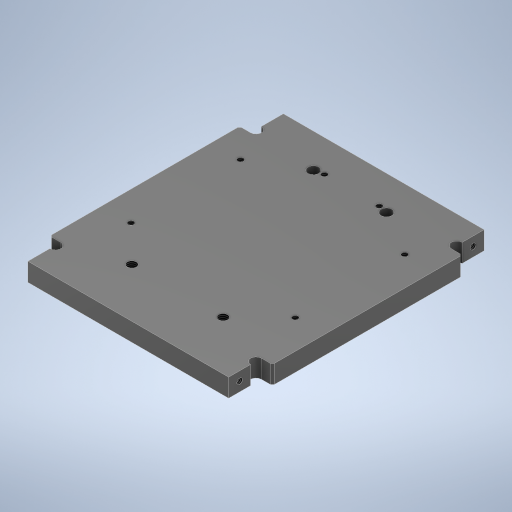
# Autodesk Inventor part: HeadCircuitMountFrame
Saved by Autodesk Inventor 2024.2 (Build 282272000, 272)
## iProperties
Created: 2024-01-19
Part Number: HeadCircuitMountFrame
Material: Acetal Resin, Black
Document SubType Name: Modeling
Designer: Masato Kubotera
Density: 1.425 g/cm^3
Appearance: Smooth - Black
Mass: 11.7532 g
Surface Area: 68.8447 cm^2
Volume: 8.24788 cm^3
Vendor: meviy
Author: Masato Kubotera
Autodesk Inventor part; units mm, degrees
ref_plane "YZ Plane" through (0, 0, 0) normal (1, 0, 0) x (0, 1, 0)
ref_plane "XZ Plane" through (0, 0, 0) normal (0, 1, 0) x (-1, 0, 0)
ref_plane "XY Plane" through (0, 0, 0) normal (0, 0, 1) x (1, 0, 0)
sketch "Sketch1" plane through (0, 0, 0) normal (0, 0, 1) x (1, 0, 0)
  line L0 (35, 27.5) -> (-35, 27.5) construction
  line L1 (-35, 27.5) -> (-35, -27.5)
  line L2 (-35, -27.5) -> (35, -27.5) construction
  line L3 (35, -27.5) -> (35, 27.5)
  line L4 (35, 27.5) -> (-35, -27.5) construction
  line L5 (-35, 27.5) -> (35, -27.5) construction
  line L6 (0, 27.5) -> (0, -27.5) construction
  line L7 (35, 0) -> (-35, 0) construction
  line L8 (26, 27.5) -> (26, 30.5)
  line L9 (26, 30.5) -> (-26, 30.5)
  line L10 (-26, 30.5) -> (-26, 27.5)
  arc A0 (-29, 27.5) -> (-26, 27.5) centre (-27.5, 27.5) ccw
  line L11 (26, -27.5) -> (26, -30.5)
  line L12 (26, -30.5) -> (-26, -30.5)
  line L13 (-26, -30.5) -> (-26, -27.5)
  arc A1 (-26, -27.5) -> (-29, -27.5) centre (-27.5, -27.5) ccw
  line L14 (-32, 27.5) -> (-32, 21.5) construction
  line L15 (0, 30.5) -> (0, 27.5) construction
  line L16 (32, 27.5) -> (32, 21.5) construction
  arc A2 (26, 27.5) -> (29, 27.5) centre (27.5, 27.5) ccw
  arc A3 (29, -27.5) -> (26, -27.5) centre (27.5, -27.5) ccw
  line L17 (-17.5, -10) -> (-35, -10) construction
  line L18 (-35, -10) -> (-35, 10) construction
  line L19 (-35, 10) -> (-17.5, 10) construction
  line L20 (-17.5, 10) -> (-17.5, -10) construction
  line L21 (-17.5, -10) -> (-35, 10) construction
  line L22 (-35, -10) -> (-17.5, 10) construction
  line L23 (-26.25, -7.5) -> (-26.25, 7.5) construction
  line L24 (-25.7386, -10) -> (-25.7386, 10) construction
  circle A4 centre (-25.7386, 10) radius 2.5 construction
  line L25 (-33, 3.75) -> (-32, 3.75)
  line L26 (-30, 1.75) -> (-30, -1.75)
  line L27 (-32, -3.75) -> (-33, -3.75)
  arc A5 (-32, -3.75) -> (-30, -1.75) centre (-32, -1.75) ccw
  arc A6 (-30, 1.75) -> (-32, 3.75) centre (-32, 1.75) ccw
  arc A7 (-35, 5.75) -> (-33, 3.75) centre (-33, 5.75) ccw
  line L28 (35, -27.5) -> (29, -27.5)
  line L29 (-29, -27.5) -> (-35, -27.5)
  line L30 (-35, 27.5) -> (-29, 27.5)
  line L31 (29, 27.5) -> (35, 27.5)
  circle A8 centre (-26.25, 7.5) radius 2.5 construction
  line L32 (14.2614, -25) -> (-20.7386, -25) construction
  line L33 (-20.7386, -25) -> (-20.7386, 25) construction
  line L34 (-20.7386, 25) -> (14.2614, 25) construction
  line L35 (14.2614, 25) -> (14.2614, -25) construction
  line L36 (14.2614, -25) -> (-20.7386, 25) construction
  line L37 (-20.7386, -25) -> (14.2614, 25) construction
  line L38 (11.7614, 22.5) -> (-18.2386, 22.5) construction
  line L39 (-18.2386, 22.5) -> (-18.2386, -22.5) construction
  line L40 (-18.2386, -22.5) -> (11.7614, -22.5) construction
  line L41 (11.7614, -22.5) -> (11.7614, 22.5) construction
  line L42 (11.7614, 22.5) -> (-18.2386, -22.5) construction
  line L43 (-18.2386, 22.5) -> (11.7614, -22.5) construction
  circle A9 centre (-18.2386, 22.5) radius 2.5 construction
  arc A10 (-21.2236, 22.2) -> (-15.2536, 22.2) centre (-18.2386, 22.5) ccw
  line L44 (-21.2386, 10) -> (-21.2386, 3)
  line L45 (-13.2637, 24) -> (6.7865, 24)
  arc A11 (8.7764, 22.2) -> (14.7464, 22.2) centre (11.7614, 22.5) ccw
  arc A12 (32.802, 10.6698) -> (32.3609, 9.408) centre (46.2004, 5.2778) ccw
  line L46 (32.9466, 11.4165) -> (32.9466, 22)
  line L47 (30.9466, 24) -> (16.7363, 24)
  arc A13 (32.802, 10.6698) -> (32.9466, 11.4165) centre (30.9466, 11.4165) ccw
  line L48 (34.9466, 11.4165) -> (32.9466, 11.4165) construction
  line L49 (32.802, 8.6698) -> (32.802, 10.6698) construction
  line L50 (30.4444, 7.9799) -> (22.1342, 7.9799)
  line L51 (15.9549, 1.8007) -> (15.9549, 3)
  line L52 (13.9549, 1) -> (-19.2386, 1)
  arc A14 (30.4444, 7.9799) -> (32.3609, 9.408) centre (30.4444, 9.9799) ccw
  arc A15 (32.9466, 22) -> (30.9466, 24) centre (30.9466, 22) ccw
  arc A16 (16.7363, 24) -> (14.7464, 22.2) centre (16.7363, 22) ccw
  arc A17 (8.7764, 22.2) -> (6.7865, 24) centre (6.7865, 22) ccw
  arc A18 (-13.2637, 24) -> (-15.2536, 22.2) centre (-13.2637, 22) ccw
  arc A19 (-21.2386, 3) -> (-19.2386, 1) centre (-19.2386, 3) ccw
  arc A20 (13.9549, 1) -> (15.9549, 3) centre (13.9549, 3) ccw
  arc A21 (22.1342, 7.9799) -> (15.9549, 1.8007) centre (22.1342, 1.8007) ccw
  arc A22 (-15.2536, -22.2) -> (-21.2236, -22.2) centre (-18.2386, -22.5) ccw
  line L53 (-21.2386, -10) -> (-21.2386, -3)
  line L54 (-13.2637, -24) -> (6.7865, -24)
  arc A23 (14.7464, -22.2) -> (8.7764, -22.2) centre (11.7614, -22.5) ccw
  arc A24 (32.3609, -9.408) -> (32.802, -10.6698) centre (46.2004, -5.2778) ccw
  line L55 (32.9466, -11.4165) -> (32.9466, -22)
  line L56 (30.9466, -24) -> (16.7363, -24)
  arc A25 (32.9466, -11.4165) -> (32.802, -10.6698) centre (30.9466, -11.4165) ccw
  line L57 (30.4444, -7.9799) -> (22.1342, -7.9799)
  line L58 (15.9549, -1.8007) -> (15.9549, -3)
  line L59 (13.9549, -1) -> (-19.2386, -1)
  arc A26 (32.3609, -9.408) -> (30.4444, -7.9799) centre (30.4444, -9.9799) ccw
  arc A27 (30.9466, -24) -> (32.9466, -22) centre (30.9466, -22) ccw
  arc A28 (14.7464, -22.2) -> (16.7363, -24) centre (16.7363, -22) ccw
  arc A29 (6.7865, -24) -> (8.7764, -22.2) centre (6.7865, -22) ccw
  arc A30 (-15.2536, -22.2) -> (-13.2637, -24) centre (-13.2637, -22) ccw
  arc A31 (-19.2386, -1) -> (-21.2386, -3) centre (-19.2386, -3) ccw
  arc A32 (15.9549, -3) -> (13.9549, -1) centre (13.9549, -3) ccw
  arc A33 (15.9549, -1.8007) -> (22.1342, -7.9799) centre (22.1342, -1.8007) ccw
  line L60 (-32.9466, 13.8893) -> (-32.9466, 22)
  arc A34 (-30.9466, 24) -> (-32.9466, 22) centre (-30.9466, 22) ccw
  arc A35 (-21.2236, 22.2) -> (-23.2135, 24) centre (-23.2135, 22) ccw
  line L61 (-30.9466, 24) -> (-23.2135, 24)
  arc A36 (-21.2386, 10) -> (-29.3442, 12.6926) centre (-25.7386, 10) ccw
  arc A37 (-32.9466, 13.8893) -> (-29.3442, 12.6926) centre (-30.9466, 13.8893) ccw
  line L62 (-32.9466, -13.8893) -> (-32.9466, -22)
  arc A38 (-32.9466, -22) -> (-30.9466, -24) centre (-30.9466, -22) ccw
  line L63 (-30.9466, -24) -> (-23.2135, -24)
  arc A39 (-29.3442, -12.6926) -> (-21.2386, -10) centre (-25.7386, -10) ccw
  arc A40 (-29.3442, -12.6926) -> (-32.9466, -13.8893) centre (-30.9466, -13.8893) ccw
  arc A41 (-23.2135, -24) -> (-21.2236, -22.2) centre (-23.2135, -22) ccw
  line L64 (25, -16) -> (-25, -16) construction
  line L65 (-25, -16) -> (-25, 16) construction
  line L66 (-25, 16) -> (25, 16) construction
  line L67 (25, 16) -> (25, -16) construction
  line L68 (25, -16) -> (-25, 16) construction
  line L69 (-25, -16) -> (25, 16) construction
  line L70 (21.5, -12.5) -> (21.5, 12.5) construction
  point P0 (0, 0)
  point P1 (0, 0)
  point P2 (0, -0.0008)
  point P3 (-29, -27.5)
  point P4 (26, -27.5)
  point P5 (-26, -27.5)
  point P6 (-26, -27.5)
  point P7 (26, -27.5)
  point P8 (-26.25, 0)
  point P9 (29, -27.5)
  point P10 (29, -10)
  point P11 (-3.2386, 0)
  point P12 (-21.2386, 22.5)
  point P13 (-15.6405, 24)
  point P14 (9.1633, 24)
  point P15 (14.3595, 24)
  point P16 (32.0128, 7.9799)
  point P17 (0, 0)
  dimension "d19" = 3
  dimension "d20" = 52
  dimension "d37" = 55
  dimension "d40" = 6
  dimension "d41" = 6
  dimension "d59" = 70
  dimension "d60" = 1.5
  dimension "d61" = 17.5
  dimension "d62" = 20
  dimension "d63" = 15
  dimension "d90" = 20
  dimension "d98" = 5
  dimension "d100" = 7.5
  dimension "d101" = 5
  dimension "d111" = 5
  dimension "d113" = 50
  dimension "d114" = 35
  dimension "d115" = 5
  dimension "d117" = 5
  dimension "d118" = 2
  dimension "d119" = 2
  dimension "d120" = 2
  dimension "d124" = 2
  dimension "d125" = 2
  dimension "d126" = 3
  dimension "d128" = 50
  dimension "d129" = 32
  dimension "d130" = 25
  dimension "d131" = 3.5
  dimension "d140" = 0
  dimension "d141" = 10
  constraints: 140 end point, 83 point on circle, 60 symmetric about line, 42 centre point, 30 tangent, 18 midpoint, 14 coincident, 14 horizontal, 11 vertical, 10 parallel, 9 point on line, 8 equal radius, 5 collinear, 5 perpendicular, 34 other
  measures "d19" distance of L8.start L8.end
  measures "d20" distance of L8.end L9.end
  measures "d37" distance of L2.end L3.end
  measures "d40" distance of L14.start L14.end
  measures "d41" distance between parallel lines of L10 L14
  measures "d59" distance of L3.end L1.start
  measures "d60" radius of A2
  measures "d61" distance of L18.end L19.end
  measures "d62" distance of L17.end L18.end
  measures "d63" distance of L23.start L23.end
  measures "d90" distance of L24.start L24.end
  measures "d98" diameter of A4
  measures "d100" distance between parallel lines of L25 L27
  measures "d101" distance between parallel lines of L26 L1
  measures "d111" diameter of A8
  measures "d113" distance of L32.end L33.end
  measures "d114" distance of L32.start L32.end
  measures "d115" distance between parallel lines of L24 L33
  measures "d117" diameter of A9
  measures "d118" distance edge to line of A4 L44
  measures "d119" radius of A13
  measures "d120" radius of A14
  measures "d124" distance edge to line of A2 L47
  measures "d125" distance between parallel lines of L52 L59
  measures "d126" radius of A11
  measures "d128" distance of L65.end L66.end
  measures "d129" distance of L64.end L65.end
  measures "d130" distance of L70.start L70.end
  measures "d131" distance between parallel lines of L67 L70
  measures "d140" distance between parallel lines of L1 L18
  measures "d141" distance between parallel lines of L1 L65
extrude "Extrusion1" add sketch "Sketch1" against normal blind 5 contours L30 A0 L10 L9 L8 A2 L31 L3 L28 A3 L11 L12 L13 A1 L29 L1 | A10 A18 L45 A17 A11 A16 L47 A15 L46 A13 A12 A14 L50 A21 L51 A20 L52 A19 L44 A36 A37 L60 A34 L61 A35 | A22 A41 L63 A38 L62 A40 A39 L53 A31 L59 A32 L58 A33 L57 A26 A24 A25 L55 A27 L56 A28 A23 A29 L54 A30
hole "M2" at (-26.25, -7.5, 0) at (-26.25, 7.5, 0) at (11.7614, 22.5, 0) at (-18.2386, 22.5, 0) at (-18.2386, -22.5, 0) at (11.7614, -22.5, 0) direction (0, 0, -1) diameter 1.567 end through all thread size "M2x0.4" class "6H" standard "ANSI Metric M Profile"
hole "Phi3" at (-25.7386, -10, 0) at (-25.7386, 10, 0) direction (0, 0, -1) diameter 3 end through all
sketch "Sketch3" plane through (29, 27.5, 0) normal (0, 1, 0) x (1, 0, 0)
  line L0 (6, 0) -> (0, 0) projected
  line L1 (3, 0) -> (3, 5)
  line L2 (-58, 0) -> (-64, 0) projected
  line L3 (-61, 0) -> (-61, 5)
  line L4 (-64, 5) -> (-58, 5) projected
  line L5 (0, 5) -> (6, 5) projected
  point P0 (-29, 0)
  point P1 (3, 0)
  point P2 (3, 2.5)
  point P3 (-61, 2.5)
  constraints: 4 end point, 4 midpoint, 2 vertical
hole "Side-M2" at (32, 27.5, -2.5) at (-32, 27.5, -2.5) direction (0, -1, 0) diameter 1.567 depth 6.3 thread size "M2x0.4" class "6H" standard "ANSI Metric M Profile"
chamfer "C0.5" distance 0.5 angle 45 4 edges at (26, -30.5, -2.5) (-26, -30.5, -2.5) (26, 30.5, -2.5) (-26, 30.5, -2.5)
mirror "Mirror1" about plane through (0, 0, 0) normal (0, 1, 0) of "Side-M2"
hole "Hole6" at (21.5, -12.5, 0) at (21.5, 12.5, 0) direction (0, 0, -1) diameter 2.459 end through all thread size "M3x0.5" class "6H" standard "ANSI Metric M Profile"
body "Solid1"
